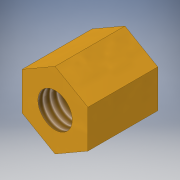
# Autodesk Inventor part: Spacer-M3-FF-05
Saved by Autodesk Inventor 2019 (Build 230136000, 136)
## iProperties
Created: 2018-04-28
Part Number: Spacer-M3-FF-05
Material: Brass, Soft Yellow, Welded
Document SubType Name: Modeling
Designer: Fierl
Density: 8.5 g/cm^3
Appearance: Weld - Brass
length: 20
Author: Fierl
Autodesk Inventor part; units mm, degrees
ref_plane "YZ Plane" through (0, 0, 0) normal (1, 0, 0) x (0, 1, 0)
ref_plane "XZ Plane" through (0, 0, 0) normal (0, 1, 0) x (-1, 0, 0)
ref_plane "XY Plane" through (0, 0, 0) normal (0, 0, 1) x (1, 0, 0)
sketch "Sketch1" plane through (0, 0, 0) normal (0, 0, 1) x (1, 0, 0)
  line L0 (2.35, 1.3568) -> (2.35, -1.3568)
  line L1 (2.35, -1.3568) -> (0, -2.7135)
  line L2 (0, -2.7135) -> (-2.35, -1.3568)
  line L3 (-2.35, 1.3568) -> (-2.35, -1.3568)
  line L4 (-2.35, 1.3568) -> (0, 2.7135)
  line L5 (0, 2.7135) -> (2.35, 1.3568)
  circle A0 centre (0, 0) radius 2.7135 construction
  line L6 (0, 29.0365) -> (0, -7.2493) construction
  line L7 (0, -14.5064) -> (0, 36.2936) projected
  line L8 (-3.799, 0) -> (3.799, 0) projected
  dimension "d0" = 5.4271
  dimension "d20" = 4.7
  dimension "d21" = 2.7136
  constraints: 14 end point, 6 point on circle, 3 coincident, 3 equal length, 2 parallel, 2 point on line, 1 centre point, 1 vertical
  measures "d0" diameter of A0
  measures "d20" distance between parallel lines of L0 L3
  measures "d21" distance of L0.start L0.end
extrude "Hexagon1" add sketch "Sketch1" along normal blind 5
hole "Hole1" at (0, 0, 0) direction (0, 0, 1) diameter 2.459 end through all thread size "M3x0.5" class "6H" standard "ISO Metric profile"
body "Solid1"
